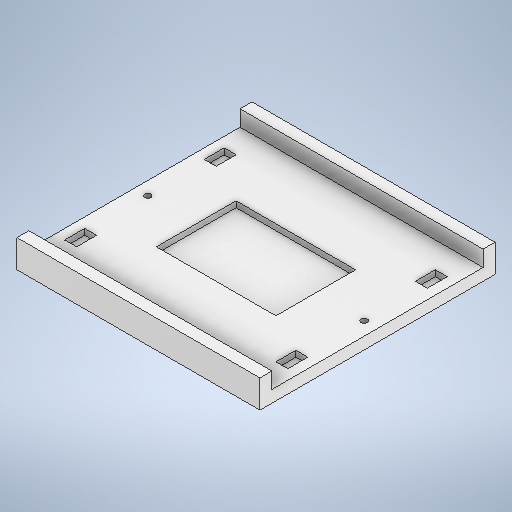
# Autodesk Inventor part: Module Holder Full V1
Saved by Autodesk Inventor 2025 (Build 290162000, 162)
## iProperties
Created: 2024-03-20
Part Number: Module Holder Full V1
Material: ABS Plastic
Document SubType Name: Modeling
Designer: cfang
Density: 1.06 g/cm^3
Appearance: Smooth - White
Author: cfang
Autodesk Inventor part; units mm, degrees
ref_plane "YZ Plane" through (0, 0, 0) normal (1, 0, 0) x (0, 1, 0)
ref_plane "XZ Plane" through (0, 0, 0) normal (0, 1, 0) x (-1, 0, 0)
ref_plane "XY Plane" through (0, 0, 0) normal (0, 0, 1) x (1, 0, 0)
sketch "Sketch1" plane through (0, 0, 0) normal (0, 1, 0) x (-1, 0, 0)
  line L0 (-30.5, -29.5) -> (30.5, -29.5)
  line L1 (30.5, -29.5) -> (30.5, 29.5)
  line L2 (30.5, 29.5) -> (-30.5, 29.5)
  line L3 (-30.5, 29.5) -> (-30.5, -29.5)
  line L4 (-30.5, -29.5) -> (30.5, 29.5) construction
  line L5 (30.5, -29.5) -> (-30.5, 29.5) construction
  point P0 (0, 0)
  dimension "d0" = 59
  dimension "d1" = 61
  constraints: 12 end point, 2 midpoint, 2 parallel, 1 horizontal, 1 perpendicular
  measures "d0" distance of L0.end L1.end
  measures "d1" distance of L1.end L2.end
extrude "Extrusion1" add sketch "Sketch1" along normal blind 7
sketch "Sketch2" plane through (0, 7, 0) normal (0, 1, 0) x (1, 0, 0)
  line L0 (-30.5, 29.5) -> (-30.5, -29.5) projected
  line L1 (30.5, 26.5) -> (-30.5, 26.5)
  line L2 (-30.5, 26.5) -> (-30.5, -26.5)
  line L3 (-30.5, -26.5) -> (30.5, -26.5)
  line L4 (30.5, -26.5) -> (30.5, 26.5)
  line L5 (30.5, 26.5) -> (-30.5, -26.5) construction
  line L6 (-30.5, 26.5) -> (30.5, -26.5) construction
  point P0 (0, 0)
  point P1 (-30.5, 26.5)
  dimension "d4" = 53
  constraints: 12 end point, 2 midpoint, 2 parallel, 1 horizontal, 1 perpendicular, 1 point on line
  measures "d4" distance between parallel lines of L3 L1
extrude "Extrusion2" cut sketch "Sketch2" against normal blind 4
sketch "Sketch3" plane through (0, 3, 0) normal (0, 1, 0) x (1, 0, 0)
  point P0 (0, 0)
  point P1 (27.15, 0)
  point P2 (-27.15, 0)
  dimension "d8" = 27.15
  dimension "d23" = 27.15
  measures "d8" distance of point (0, 0) point (27.15, 0)
  measures "d23" distance of point (0, 0) point (-27.15, 0)
hole "Hole1" at (27.15, 3, 0) at (-27.15, 3, 0) direction (0, -1, 0) diameter 1.567 end through all thread size "M2x0.4" class "6H" standard "ANSI Metric M Profile"
sketch "Sketch5" plane through (0, 3, 0) normal (0, 1, 0) x (1, 0, 0)
  line L0 (15, -10) -> (-15, -10)
  line L1 (-15, -10) -> (-15, 10)
  line L2 (-15, 10) -> (15, 10)
  line L3 (15, 10) -> (15, -10)
  line L4 (15, -10) -> (-15, 10) construction
  line L5 (-15, -10) -> (15, 10) construction
  line L6 (-28, 20) -> (-25, 20)
  line L7 (-25, 20) -> (-25, 15)
  line L8 (-25, 15) -> (-28, 15)
  line L9 (-28, 15) -> (-28, 20)
  line L10 (-28, 20) -> (-25, 15) construction
  line L11 (-25, 20) -> (-28, 15) construction
  line L12 (-28, -15) -> (-25, -15)
  line L13 (-25, -15) -> (-25, -20)
  line L14 (-25, -20) -> (-28, -20)
  line L15 (-28, -20) -> (-28, -15)
  line L16 (-28, -15) -> (-25, -20) construction
  line L17 (-25, -15) -> (-28, -20) construction
  line L18 (25, -15) -> (28, -15)
  line L19 (28, -15) -> (28, -20)
  line L20 (28, -20) -> (25, -20)
  line L21 (25, -20) -> (25, -15)
  line L22 (25, -15) -> (28, -20) construction
  line L23 (28, -15) -> (25, -20) construction
  line L24 (25, 20) -> (28, 20)
  line L25 (28, 20) -> (28, 15)
  line L26 (28, 15) -> (25, 15)
  line L27 (25, 15) -> (25, 20)
  line L28 (25, 20) -> (28, 15) construction
  line L29 (28, 20) -> (25, 15) construction
  point P0 (0, 0)
  point P1 (-26.5, 17.5)
  point P2 (-26.5, -17.5)
  point P3 (26.5, -17.5)
  point P4 (26.5, 17.5)
  point P5 (-25, 17.5)
  dimension "d24" = 30
  dimension "d25" = 20
  dimension "d26" = 5
  dimension "d27" = 3
  dimension "d28" = 5
  dimension "d29" = 3
  dimension "d30" = 5
  dimension "d31" = 3
  dimension "d32" = 5
  dimension "d33" = 3
  dimension "d35" = 25
  dimension "d36" = 15
  dimension "d38" = 25
  dimension "d39" = 15
  constraints: 60 end point, 11 midpoint, 10 parallel, 5 horizontal, 5 perpendicular, 2 horizontal alignment, 2 vertical alignment
  measures "d24" distance of L1.end L2.end
  measures "d25" distance of L0.end L1.end
  measures "d26" distance of L6.end L7.end
  measures "d27" distance of L7.end L8.end
  measures "d28" distance of L12.end L13.end
  measures "d29" distance of L13.end L14.end
  measures "d30" distance of L26.end L24.start
  measures "d31" distance of L25.end L26.end
  measures "d32" distance of L20.end L18.start
  measures "d33" distance of L18.start L18.end
  measures "d35" distance from line of L7 point (0, 0)
  measures "d36" distance from line of point (0, 0) L8
  measures "d38" distance from line of L27 point (0, 0)
  measures "d39" distance from line of L12 point (0, 0)
extrude "Extrusion4" cut sketch "Sketch5" against normal blind 1.5
equation "\"d8\" = d7"
equation "\"d23\" = d8"
equation "\"d28\" = d26"
equation "\"d29\" = d27"
equation "\"d30\" = d26"
equation "\"d31\" = d27"
equation "\"d32\" = d26"
equation "\"d33\" = d27"
equation "\"d38\" = d35"
equation "\"d39\" = d36"
equation "\"d7\" = 27.15"
body "Solid1"
